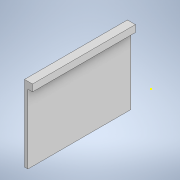
# Autodesk Inventor part: Part2
Saved by Autodesk Inventor 2022 (Build 260153000, 153)
## iProperties
Created: 2022-04-28
Part Number: Part2
Material: Generic
Document SubType Name: Modeling
Designer: Oana
Density: 1 g/cm^3
Appearance: Default
Author: Oana
Autodesk Inventor part; units mm, degrees
ref_plane "YZ Plane" through (0, 0, 0) normal (1, 0, 0) x (0, 1, 0)
ref_plane "XZ Plane" through (0, 0, 0) normal (0, 1, 0) x (-1, 0, 0)
ref_plane "XY Plane" through (0, 0, 0) normal (0, 0, 1) x (1, 0, 0)
sketch "Sketch1" plane through (0, 0, 0) normal (1, 0, 0) x (0, 1, 0)
  line L0 (59.5474, 107.5539) -> (-6.8486, 107.5539)
  line L1 (-6.8486, 107.5539) -> (-6.8486, 17.5539)
  line L2 (-6.8486, 17.5539) -> (59.5474, 17.5539)
  line L3 (59.5474, 17.5539) -> (59.5474, 107.5539)
  point P0 (0, 0)
  dimension "d0" = 90
  dimension "d1" = 66.396
  constraints: 8 end point, 2 parallel, 1 horizontal, 1 perpendicular
  measures "d0" distance of L2.end L0.start
  measures "d1" distance of L1.end L2.end
extrude "Extrusion1" add sketch "Sketch1" along normal blind 3
sketch "Sketch2" plane through (3, 0, 0) normal (1, 0, 0) x (0, 0, -1)
  point P0 (0, 0)
sketch "Sketch3" plane through (3, 0, 0) normal (1, 0, 0) x (0, 0, -1)
  line L0 (-107.5539, -6.8486) -> (-17.5539, -6.8486) projected
  line L1 (-17.5539, -6.8486) -> (-17.5539, 59.5474) projected
  line L2 (-17.5539, 59.5474) -> (-107.5539, 59.5474) projected
  line L3 (-107.5539, 59.5474) -> (-107.5539, -6.8486) projected
  line L4 (-107.5539, 59.5474) -> (-17.5539, 59.5474)
  line L5 (-17.5539, 59.5474) -> (-17.5539, 53.5474)
  line L6 (-17.5539, 53.5474) -> (-107.5539, 53.5474)
  line L7 (-107.5539, 53.5474) -> (-107.5539, 59.5474)
  point P0 (0, 0)
  dimension "d4" = 6
  constraints: 8 end point, 2 parallel, 1 horizontal, 1 perpendicular, 1 point on line
  measures "d4" distance between parallel lines of L2 L6
extrude "Extrusion2" add sketch "Sketch3" along normal blind 4 contours L3 L2 L1 L6
body "Solid1"
